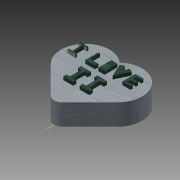
# Autodesk Inventor part: Herz
Saved by Autodesk Inventor 2015 (Build 190159000, 159)
## iProperties
Created: 2017-06-28
Part Number: Herz
Material: Generisch
Document SubType Name: Modeling
Designer: s0554918
Density: 1 g/cm^3
Appearance: Vorgabe
Author: s0554918
Autodesk Inventor part; units mm, degrees
ref_plane "YZ Plane" through (0, 0, 0) normal (1, 0, 0) x (0, 1, 0)
ref_plane "XZ Plane" through (0, 0, 0) normal (0, 1, 0) x (-1, 0, 0)
ref_plane "XY Plane" through (0, 0, 0) normal (0, 0, 1) x (1, 0, 0)
sketch "Skizze1" plane through (0, 0, 0) normal (0, 0, 1) x (1, 0, 0)
  arc A0 (20.6066, -0.6066) -> (0, 21.1803) centre (10, 10) ccw
  line L0 (-43.6814, 0) -> (43.6814, 0) projected
  line L1 (0, -31.696) -> (0, 41.6836) projected
  line L2 (-20.6066, -0.6066) -> (-3.5355, -17.6777)
  line L3 (20.6066, -0.6066) -> (3.5355, -17.6777)
  arc A1 (-3.5355, -17.6777) -> (3.5355, -17.6777) centre (0, -14.1421) ccw
  arc A2 (0, 21.1803) -> (-20.6066, -0.6066) centre (-10, 10) ccw
  point P0 (0, 0)
  point P1 (0, -21.2132)
  dimension "d0" = 10
  dimension "d2" = 10
  dimension "d3" = 30
  dimension "d4" = 10
  dimension "d5" = 10
  dimension "d6" = 5
  dimension "d7" = 45
  dimension "d8" = 45
  constraints: 6 point on circle, 4 end point, 4 tangent, 3 centre point, 3 point on line
  measures "d0" distance from line of L1 A2.centre
  measures "d2" distance from line of L1 A0.centre
  measures "d3" diameter of A0
  measures "d4" distance from line of L0 A2.centre
  measures "d5" distance from line of L0 A0.centre
  measures "d6" radius of A1
  measures "d7" angle of L1 L2
  measures "d8" angle of L1 L3
extrude "Extrusion1" add sketch "Skizze1" along normal blind 15
sketch "Skizze2" plane through (0, 0, 15) normal (0, 0, 1) x (1, 0, 0)
  line L0 (-19, 17) -> (-19, 11)
  line L1 (-19, 11) -> (-21, 11)
  line L2 (-21, 11) -> (-21, 10)
  line L3 (-21, 10) -> (-16, 10)
  line L4 (-16, 10) -> (-16, 11)
  line L5 (-16, 11) -> (-18, 11)
  line L6 (-18, 11) -> (-18, 17)
  line L7 (-18, 17) -> (-16, 17)
  line L8 (-16, 17) -> (-16, 18)
  line L9 (-16, 18) -> (-21, 18)
  line L10 (-21, 18) -> (-21, 17)
  line L11 (-21, 17) -> (-19, 17)
  line L12 (-20.6066, -0.6066) -> (-3.5355, -17.6777) projected
  arc A0 (-3.5355, -17.6777) -> (3.5355, -17.6777) centre (0, -14.1421) ccw projected
  line L13 (3.5355, -17.6777) -> (20.6066, -0.6066) projected
  arc A1 (20.6066, -0.6066) -> (0, 21.1803) centre (10, 10) ccw projected
  arc A2 (0, 21.1803) -> (-20.6066, -0.6066) centre (-10, 10) ccw projected
  line L14 (-10, 18) -> (-10, 10)
  line L15 (-10, 10) -> (-4, 10)
  line L16 (-4, 10) -> (-4, 12)
  line L17 (-4, 12) -> (-9, 12)
  line L18 (-9, 12) -> (-9, 18)
  line L19 (-9, 18) -> (-10, 18)
  line L20 (-1.8657, 18) -> (-1.8657, 10)
  line L21 (-1.8657, 10) -> (1.8657, 10)
  line L22 (1.8657, 10) -> (1.8657, 18)
  line L23 (1.8657, 18) -> (-1.8657, 18)
  line L24 (-1, 16) -> (-1, 12)
  line L25 (-1, 12) -> (1, 12)
  line L26 (1, 12) -> (1, 16)
  line L27 (1, 16) -> (-1, 16)
  line L28 (12.8657, 16) -> (12.8657, 10)
  line L29 (12.8657, 10) -> (17.8657, 10)
  line L30 (17.8657, 10) -> (17.8657, 11.3333)
  line L31 (17.8657, 11.3333) -> (14.8657, 11.3333)
  line L32 (14.8657, 11.3333) -> (14.8657, 13.3333)
  line L33 (14.8657, 13.3333) -> (17.8657, 13.3333)
  line L34 (17.8657, 13.3333) -> (17.8657, 14.6667)
  line L35 (17.8657, 14.6667) -> (14.8657, 14.6667)
  line L36 (14.8657, 14.6667) -> (14.8657, 16.6667)
  line L37 (14.8657, 16.6667) -> (17.8657, 16.6667)
  line L38 (17.8657, 16.6667) -> (17.8657, 18)
  line L39 (17.8657, 18) -> (12.8657, 18)
  line L40 (12.8657, 18) -> (12.8657, 14.6667)
  line L41 (-4, 3.5) -> (-4, -3.5)
  line L42 (-6, -3.5) -> (-6, 3.5)
  line L43 (-8, 5.5) -> (-2, 5.5)
  line L44 (-2, 5.5) -> (-2, 3.5)
  line L45 (-8, 3.5) -> (-8, 5.5)
  line L46 (-2, -3.5) -> (-2, -5.5)
  line L47 (-2, -5.5) -> (-8, -5.5)
  line L48 (-8, -5.5) -> (-8, -3.5)
  line L49 (-43.6814, 0) -> (43.6814, 0) projected
  line L50 (0, -29.2107) -> (0, 41.2693) projected
  line L51 (3.1352, 18) -> (6.8657, 10)
  line L52 (6.8657, 10) -> (10.5961, 18)
  line L53 (10.5961, 18) -> (8.4516, 19)
  line L54 (8.4516, 19) -> (6.8657, 15.5989)
  line L55 (6.8657, 15.5989) -> (5.2797, 19)
  line L56 (5.2797, 19) -> (3.1352, 18)
  line L57 (-2, 3.5) -> (-4, 3.5)
  line L58 (-6, 3.5) -> (-8, 3.5)
  line L59 (-8, -3.5) -> (-6, -3.5)
  line L60 (-4, -3.5) -> (-2, -3.5)
  line L61 (4, 3.5) -> (4, -3.5)
  line L62 (6, -3.5) -> (6, 3.5)
  line L63 (8, 5.5) -> (2, 5.5)
  line L64 (2, 5.5) -> (2, 3.5)
  line L65 (8, 3.5) -> (8, 5.5)
  line L66 (2, -3.5) -> (2, -5.5)
  line L67 (2, -5.5) -> (8, -5.5)
  line L68 (8, -5.5) -> (8, -3.5)
  line L69 (2, 3.5) -> (4, 3.5)
  line L70 (6, 3.5) -> (8, 3.5)
  line L71 (8, -3.5) -> (6, -3.5)
  line L72 (4, -3.5) -> (2, -3.5)
  dimension "d11" = 2
  dimension "d12" = 10
  dimension "d14" = 10
  dimension "d15" = 8
  dimension "d16" = 8
  dimension "d17" = 1
  dimension "d18" = 4
  dimension "d19" = 4
  dimension "d20" = 1.8657
  dimension "d21" = 2
  dimension "d22" = 1
  dimension "d23" = 6
  dimension "d24" = 2
  dimension "d26" = 10
  dimension "d27" = 50
  dimension "d28" = 50
  dimension "d29" = 5
  dimension "d30" = 8
  dimension "d31" = 8
  dimension "d32" = 9
  dimension "d33" = 9
  dimension "d34" = 8
  dimension "d35" = 6
  dimension "d36" = 5
  dimension "d37" = 2
  dimension "d38" = 2
  dimension "d39" = 90
  dimension "d40" = 2
  dimension "d41" = 2
  dimension "d42" = 2
  dimension "d43" = 7
  constraints: 138 end point, 32 perpendicular, 19 point on line, 18 equal length, 12 symmetric about line, 7 parallel, 3 horizontal, 3 vertical, 5 other
  measures "d11" distance of L4.end L5.end
  measures "d12" distance between parallel lines of L49 L3
  measures "d14" distance between parallel lines of L49 L29
  measures "d15" distance between parallel lines of L3 L9
  measures "d16" distance of L14.start L14.end
  measures "d17" distance of L18.end L14.start
  measures "d18" distance of L24.start L24.end
  measures "d19" distance from line of L50 L15.end
  measures "d20" distance between parallel lines of L20 L50
  measures "d21" distance between parallel lines of L23 L27
  measures "d22" distance between parallel lines of L6 L0
  measures "d23" distance of L14.end L3.end
  measures "d24" distance of L26.end L24.start
  measures "d26" distance from line of L49 L51.end
  measures "d27" angle of L52 L51
  measures "d28" angle of L54 L55
  measures "d29" distance of L51.end L21.end
  measures "d30" distance from line of L21 L51.start
  measures "d31" distance from line of L21 L52.end
  measures "d32" distance from line of L21 L55.end
  measures "d33" distance from line of L21 L53.end
  measures "d34" distance of L28.end L39.end
  measures "d35" distance of L28.end L51.end
  measures "d36" distance of L38.end L39.end
  measures "d37" distance of L35.end L36.end
  measures "d38" distance from line of L28 L31.end
  measures "d39" angle of L42 L58
  measures "d40" distance of L43.end L44.end
  measures "d41" distance between parallel lines of L41 L42
  measures "d42" distance from line of L50 L46.end
  measures "d43" distance of L42.start L42.end
extrude "Extrusion2" cut sketch "Skizze2" against normal blind 2 contours A2 L49 L42 L59 L48 L47 L46 L60 L41 L50 A0 L12 | A2 L50 L23 L20 L21 L49 L41 L57 L44 L43 L45 L58 L42 | L50 L49 L61 L72 L66 L67 L68 L71 L62 A1 L13 A0 | A1 L49 L62 L70 L65 L63 L64 L69 L61 L50 L21 L22 L23
